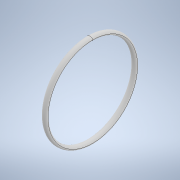
# Autodesk Inventor part: neumatico
Saved by Autodesk Inventor 2021 (Build 250183000, 183)
## iProperties
Created: 2021-04-15
Part Number: neumatico
Material: Genérico
Document SubType Name: Modeling
Designer: j2seb
Density: 1 g/cm^3
Appearance: Valor por defecto
Author: j2seb
Autodesk Inventor part; units mm, degrees
note: some values were not read from the file. Chosen so that the rebuilt part matches the saved one: offset side.
ref_plane "YZ Plane" through (0, 0, 0) normal (1, 0, 0) x (0, 1, 0)
ref_plane "XZ Plane" through (0, 0, 0) normal (0, 1, 0) x (-1, 0, 0)
ref_plane "XY Plane" through (0, 0, 0) normal (0, 0, 1) x (1, 0, 0)
sketch "Boceto1" plane through (0, 0, 0) normal (0, 0, 1) x (1, 0, 0)
  spline S0 degree 4 poles (-24.9404, 274.1789) (-12.6331, 270.0547) (0, 268.534) (12.6331, 270.0547) (24.9404, 274.1789) knots 0 0 0 0 0 1 1 1 1 1
  line L0 (-27.5011, 282.6709) -> (-27.5011, 0)
  line L1 (27.5011, 0) -> (27.5011, 282.6709)
  ellipse E0 centre (0, 290) end of major axis (18, 290) minor radius 12
  line L2 (-27.5011, 0) -> (27.5011, 0)
  spline S1 degree 5 poles (15, 290) (15.0003, 290.7435) (14.8607, 291.4892) (14.586, 292.1936) (13.7106, 293.7608) (12.431, 295.0357) (11.6096, 295.6815) (9.6167, 296.9617) (7.4175, 297.8506) (6.1508, 298.2419) (3.4643, 298.8509) (0.7159, 299.0527) (-0.7158, 299.0527) (-3.4642, 298.8509) (-6.1508, 298.242) (-7.4175, 297.8505) (-9.6168, 296.9618) (-11.6097, 295.6814) (-12.431, 295.0359) (-13.7108, 293.7603) (-14.586, 292.1939) (-14.861, 291.4881) (-15.1391, 290) (-14.861, 288.5119) (-14.586, 287.8061) (-13.7108, 286.2397) (-12.431, 284.9641) (-11.6097, 284.3186) (-9.6168, 283.0382) (-7.4175, 282.1495) (-6.1508, 281.758) (-3.4642, 281.1491) (-0.7158, 280.9473) (0.7159, 280.9473) (3.4643, 281.1491) (6.1508, 281.7581) (7.4175, 282.1494) (9.6167, 283.0383) (11.6096, 284.3185) (12.431, 284.9643) (13.7106, 286.2392) (14.586, 287.8064) (14.8607, 288.5108) (15.0003, 289.2565) (15, 290) knots 0 0 0 0 0 0 0.048716 0.048716 0.048716 0.116783 0.116783 0.116783 0.203271 0.203271 0.203271 0.296728 0.296728 0.296728 0.383218 0.383218 0.383218 0.451287 0.451287 0.451287 0.5 0.5 0.5 0.548713 0.548713 0.548713 0.616782 0.616782 0.616782 0.703272 0.703272 0.703272 0.796729 0.796729 0.796729 0.883217 0.883217 0.883217 0.951284 0.951284 0.951284 1 1 1 1 1 1
  point P0 (0, 0)
  point P1 (-12.4232, 271.0369)
  point P2 (0, 270)
  point P3 (12.4232, 271.0369)
  dimension "d0" = 18
  dimension "d1" = 12
  dimension "d2" = 290
  dimension "d4" = 3
  constraints: 6 end point, 1 centre point, 1 horizontal, 1 vertical alignment, 6 other
  measures "d2" distance of point (0, 0) E0.centre
revolve "Revolución1" add sketch "Boceto1" angle 360 about axis through (-27.5011, 0, 0) along (1, 0, 0)
